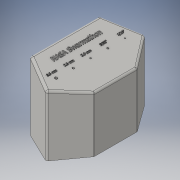
# Autodesk Inventor part: HexKeyStand
Saved by Autodesk Inventor 2016 (Build 200138000, 138)
## iProperties
Created: 2016-07-28
Part Number: HexKeyStand
Material: Generic
Document SubType Name: Modeling
Designer: lachesis
Density: 1 g/cm^3
Appearance: Default
Author: lachesis
Autodesk Inventor part; units mm, degrees
(part 1 of 3)
ref_plane "YZ Plane" through (0, 0, 0) normal (1, 0, 0) x (0, 1, 0)
ref_plane "XZ Plane" through (0, 0, 0) normal (0, 1, 0) x (-1, 0, 0)
ref_plane "XY Plane" through (0, 0, 0) normal (0, 0, 1) x (1, 0, 0)
sketch "Sketch1" plane through (0, 0, 0) normal (0, 1, 0) x (-1, 0, 0)
  line L0 (-29.7389, 31.75) -> (-29.7389, -31.75)
  line L1 (-29.7389, -31.75) -> (0, -72.9354)
  line L2 (0, -72.9354) -> (45.7238, -50.8)
  line L3 (45.7238, -50.8) -> (45.7238, 50.8)
  line L4 (45.7238, 50.8) -> (0, 72.9354)
  line L5 (0, 72.9354) -> (-29.7389, 31.75)
  point P0 (0, 0)
  point P1 (45.7238, 0)
  point P2 (-29.7389, 0)
  dimension "d0" = 101.6
  dimension "d1" = 63.5
  dimension "d2" = 50.8
  dimension "d3" = 50.8
  dimension "d5" = 50.8
  dimension "d6" = 100
  constraints: 12 end point, 2 horizontal alignment, 2 midpoint, 2 vertical alignment, 1 parallel, 1 vertical
  measures "d0" distance of L2.end L3.end
  measures "d1" distance of L0.start L0.end
  measures "d2" distance of L3.end L4.end
  measures "d3" distance of L1.end L2.end
  measures "d5" distance of L4.end L0.start
  measures "d6" angle of L1 L2
extrude "Extrusion1" add sketch "Sketch1" along normal blind 101.6
ref_plane "Work Plane4" through (0, 0, 72.9354) normal (0, 0, -1) x (0, 1, 0)
ref_plane "Work Plane3" through (29.7389, 0, 31.75) normal (0, 0, -1) x (0, 1, 0)
sketch "Sketch3" plane through (0, 0, 72.9354) normal (0, 0, -1) x (0, 1, 0)
  line L0 (0, -45.7238) -> (101.6, -45.7238) projected
  line L1 (101.6, -45.7238) -> (101.6, 0) projected
  line L2 (101.6, 0) -> (101.6, 29.7389) projected
  line L3 (0, 29.7389) -> (101.6, 29.7389) projected
  line L4 (0, -45.7238) -> (101.6, -45.7238) projected
  line L5 (101.6, -45.7238) -> (81.3798, 29.7389)
  point P0 (0, 0)
  dimension "d14" = 15
  constraints: 2 end point, 1 point on line
  measures "d14" angle of L1 L5
extrude "Extrusion3" cut sketch "Sketch3" along normal through all
fillet "Fillet1" radius 3.175 12 edges at (-22.8619, 95.4742, 61.8677) (-45.7238, 101.6, 0) (-45.7238, 50.8, 50.8) (0, 44.6742, 72.9354) (29.7389, 40.6899, 31.75) (14.8695, 85.3641, 52.3427) (29.7389, 81.3798, 0) (29.7389, 40.6899, -31.75) (14.8695, 85.3641, -52.3427) (0, 44.6742, -72.9354) (-22.8619, 95.4742, -61.8677) (-45.7238, 50.8, -50.8)
sketch "Sketch4" plane through (-41.727, 100.5291, 48.8096) normal (0.258819, 0.9659258, 0) x (0.9659258, -0.258819, 0)
  line L0 (0, 0) -> (0, 97.6191) projected
  line L1 (0, 48.8096) -> (71.5508, 48.8096)
  line L2 (71.5508, 79.5331) -> (71.5508, 18.086) projected
  line L3 (35.7754, 48.8096) -> (35.7754, 127.794)
  line L4 (35.7754, 127.794) -> (35.7754, 48.8096)
  line L5 (35.7754, 48.8096) -> (35.7754, -35.2396)
  line L6 (35.7754, 24.8529) -> (37.0254, 24.1313)
  line L7 (37.0254, 24.1313) -> (37.0254, 22.6879)
  line L8 (37.0254, 22.6879) -> (35.7754, 21.9662)
  line L9 (35.7754, 21.9662) -> (34.5254, 22.6879)
  line L10 (34.5254, 22.6879) -> (34.5254, 24.1313)
  line L11 (34.5254, 24.1313) -> (35.7754, 24.8529)
  line L12 (35.7754, 49.9643) -> (36.7754, 49.3869)
  line L13 (36.7754, 49.3869) -> (36.7754, 48.2322)
  line L14 (36.7754, 48.2322) -> (35.7754, 47.6549)
  line L15 (35.7754, 47.6549) -> (34.7754, 48.2322)
  line L16 (34.7754, 48.2322) -> (34.7754, 49.3869)
  line L17 (34.7754, 49.3869) -> (35.7754, 49.9643)
  line L18 (35.7754, 75.5844) -> (36.966, 74.897)
  line L19 (36.966, 74.897) -> (36.966, 73.5222)
  line L20 (36.966, 73.5222) -> (35.7754, 72.8348)
  line L21 (35.7754, 72.8348) -> (34.5848, 73.5222)
  line L22 (34.5848, 73.5222) -> (34.5848, 74.897)
  line L23 (34.5848, 74.897) -> (35.7754, 75.5844)
  line L24 (35.7754, 98.693) -> (34.9816, 99.1513)
  line L25 (34.9816, 99.1513) -> (34.9816, 100.0678)
  line L26 (34.9816, 100.0678) -> (35.7754, 100.5261)
  line L27 (35.7754, 100.5261) -> (36.5691, 100.0678)
  line L28 (36.5691, 100.0678) -> (36.5691, 99.1513)
  line L29 (36.5691, 99.1513) -> (35.7754, 98.693)
  line L30 (35.7754, 0.0303) -> (37.5254, -0.9801)
  line L31 (37.5254, -0.9801) -> (37.5254, -3.0008)
  line L32 (37.5254, -3.0008) -> (35.7754, -4.0112)
  line L33 (35.7754, -4.0112) -> (34.0254, -3.0008)
  line L34 (34.0254, -3.0008) -> (34.0254, -0.9801)
  line L35 (34.0254, -0.9801) -> (35.7754, 0.0303)
  point P0 (66.3241, 48.8096)
  point P1 (35.7754, -1.9904)
  point P2 (35.7754, 23.4096)
  point P3 (35.7754, 74.2096)
  point P4 (35.7754, 99.6096)
  point P5 (35.7754, -1.9904)
  point P6 (35.7754, 23.4096)
  point P7 (35.7754, 74.2096)
  point P8 (35.7754, 99.6096)
  point P9 (35.7754, -1.9904)
  dimension "d18" = 25.4
  dimension "d19" = 25.4
  dimension "d20" = 25.4
  dimension "d22" = 25.4
  dimension "d23" = 3.5
  dimension "d24" = 2.5
  dimension "d25" = 2
  dimension "d26" = 2.3813
  dimension "d27" = 1.5875
  constraints: 68 end point, 9 point on line, 6 coincident, 3 midpoint, 2 vertical, 1 perpendicular, 65 other
  measures "d18" distance of point (35.775, 74.21) L3.start
  measures "d19" distance of point (35.775, 74.21) point (35.775, 99.61)
  measures "d20" distance of L3.start point (35.775, 23.41)
  measures "d22" distance of point (35.775, 23.41) point (35.775, -1.99)
  measures "d23" distance between parallel lines of L31 L34
  measures "d24" distance between parallel lines of L7 L10
  measures "d25" distance between parallel lines of L13 L16
  measures "d26" distance between parallel lines of L19 L22
  measures "d27" distance between parallel lines of L28 L25
extrude "Extrusion4" cut sketch "Sketch4" against normal blind 76.2
sketch "Sketch5" plane through (-41.727, 100.5291, 48.8096) normal (0.258819, 0.9659258, 0) x (0.9659258, -0.258819, 0)
  line L0 (34.0254, -3.0008) -> (34.0254, -0.9801) projected
  spline S0 degree 2 poles (26.7586, -7.3009) (26.7586, -7.412) (26.8129, -7.6319) (26.8549, -7.7381) knots 0 0 0 1 2 2 2
  spline S1 degree 2 poles (26.8549, -7.7381) (26.8969, -7.8369) (26.9858, -7.9826) (27.0254, -8.0394) knots 0 0 0 1 2 2 2
  line L1 (27.0254, -8.0394) -> (27.0254, -8.0641)
  line L2 (27.0254, -8.0641) -> (26.5931, -8.0641)
  spline S2 degree 2 poles (26.5931, -8.0641) (26.5215, -7.9307) (26.4054, -7.4738) (26.4054, -7.2688) knots 0 0 0 1 2 2 2
  spline S3 degree 2 poles (26.4054, -7.2688) (26.4054, -7.0613) (26.4894, -6.7525) (26.5783, -6.6266) knots 0 0 0 1 2 2 2
  spline S4 degree 2 poles (26.5783, -6.6266) (26.6746, -6.4932) (26.9537, -6.3549) (27.1414, -6.3549) knots 0 0 0 1 2 2 2
  spline S5 degree 2 poles (27.1414, -6.3549) (27.3934, -6.3549) (27.7738, -6.6858) (27.8232, -6.918) knots 0 0 0 1 2 2 2
  line L3 (27.8232, -6.918) -> (27.8528, -6.918)
  spline S6 degree 2 poles (27.8528, -6.918) (27.8726, -6.8217) (27.9615, -6.6019) (28.0504, -6.508) knots 0 0 0 1 2 2 2
  spline S7 degree 2 poles (28.0504, -6.508) (28.1369, -6.4141) (28.4135, -6.2956) (28.6136, -6.2956) knots 0 0 0 1 2 2 2
  spline S8 degree 2 poles (28.6136, -6.2956) (28.8186, -6.2956) (29.1669, -6.4364) (29.3002, -6.5648) knots 0 0 0 1 2 2 2
  spline S9 degree 2 poles (29.3002, -6.5648) (29.4386, -6.6982) (29.5818, -7.0761) (29.5818, -7.3157) knots 0 0 0 1 2 2 2
  spline S10 degree 2 poles (29.5818, -7.3157) (29.5818, -7.5454) (29.4707, -7.9949) (29.3941, -8.1481) knots 0 0 0 1 2 2 2
  line L4 (29.3941, -8.1481) -> (28.9619, -8.1481)
  line L5 (28.9619, -8.1481) -> (28.9619, -8.1184)
  spline S11 degree 2 poles (28.9619, -8.1184) (29.0557, -7.99) (29.2286, -7.5553) (29.2286, -7.3404) knots 0 0 0 1 2 2 2
  spline S12 degree 2 poles (29.2286, -7.3404) (29.2286, -7.2144) (29.1496, -6.9625) (29.0582, -6.8785) knots 0 0 0 1 2 2 2
  spline S13 degree 2 poles (29.0582, -6.8785) (28.9668, -6.797) (28.7494, -6.7105) (28.5839, -6.7105) knots 0 0 0 1 2 2 2
  spline S14 degree 2 poles (28.5839, -6.7105) (28.4184, -6.7105) (28.2036, -6.8069) (28.1418, -6.8933) knots 0 0 0 1 2 2 2
  spline S15 degree 2 poles (28.1418, -6.8933) (28.0801, -6.9798) (28.0331, -7.2144) (28.0331, -7.3527) knots 0 0 0 1 2 2 2
  line L6 (28.0331, -7.3527) -> (28.0331, -7.5256)
  line L7 (28.0331, -7.5256) -> (27.6947, -7.5256)
  line L8 (27.6947, -7.5256) -> (27.6947, -7.3898)
  spline S16 degree 2 poles (27.6947, -7.3898) (27.6947, -7.1156) (27.4329, -6.7698) (27.1834, -6.7698) knots 0 0 0 1 2 2 2
  spline S17 degree 2 poles (27.1834, -6.7698) (27.0673, -6.7698) (26.9019, -6.8587) (26.8525, -6.9304) knots 0 0 0 1 2 2 2
  spline S18 degree 2 poles (26.8525, -6.9304) (26.8006, -7.0069) (26.7586, -7.1947) (26.7586, -7.3009) knots 0 0 0 1 2 2 2
  line L9 (29.5176, -5.1816) -> (29.5176, -5.6707)
  line L10 (29.5176, -5.6707) -> (28.9347, -5.6707)
  line L11 (28.9347, -5.6707) -> (28.9347, -5.1816)
  line L12 (28.9347, -5.1816) -> (29.5176, -5.1816)
  spline S19 degree 2 poles (28.5494, -2.719) (28.7692, -2.719) (29.1446, -2.8598) (29.283, -2.9882) knots 0 0 0 1 2 2 2
  spline S20 degree 2 poles (29.283, -2.9882) (29.4213, -3.1167) (29.5818, -3.4995) (29.5818, -3.7366) knots 0 0 0 1 2 2 2
  spline S21 degree 2 poles (29.5818, -3.7366) (29.5818, -3.954) (29.4855, -4.3788) (29.4089, -4.5345) knots 0 0 0 1 2 2 2
  line L13 (29.4089, -4.5345) -> (28.9767, -4.5345)
  line L14 (28.9767, -4.5345) -> (28.9767, -4.5048)
  spline S22 degree 2 poles (28.9767, -4.5048) (29.0113, -4.4579) (29.1002, -4.2825) (29.1397, -4.1763) knots 0 0 0 1 2 2 2
  spline S23 degree 2 poles (29.1397, -4.1763) (29.1817, -4.0553) (29.2286, -3.8552) (29.2286, -3.7292) knots 0 0 0 1 2 2 2
  spline S24 degree 2 poles (29.2286, -3.7292) (29.2286, -3.6057) (29.1397, -3.3735) (29.0434, -3.2896) knots 0 0 0 1 2 2 2
  spline S25 degree 2 poles (29.0434, -3.2896) (28.952, -3.213) (28.7099, -3.134) (28.5469, -3.134) knots 0 0 0 1 2 2 2
  spline S26 degree 2 poles (28.5469, -3.134) (28.3839, -3.134) (28.1764, -3.2229) (28.1072, -3.3069) knots 0 0 0 1 2 2 2
  spline S27 degree 2 poles (28.1072, -3.3069) (28.0307, -3.3933) (27.9664, -3.6502) (27.9664, -3.8058) knots 0 0 0 1 2 2 2
  spline S28 degree 2 poles (27.9664, -3.8058) (27.9664, -3.9738) (28.0183, -4.3072) (28.0405, -4.4085) knots 0 0 0 1 2 2 2
  line L15 (28.0405, -4.4085) -> (26.4696, -4.4085)
  line L16 (26.4696, -4.4085) -> (26.4696, -2.7363)
  line L17 (26.4696, -2.7363) -> (26.8278, -2.7363)
  line L18 (26.8278, -2.7363) -> (26.8278, -4.0158)
  line L19 (26.8278, -4.0158) -> (27.6404, -4.0158)
  spline S29 degree 2 poles (27.6404, -4.0158) (27.6305, -3.9417) (27.6231, -3.7984) (27.6231, -3.7391) knots 0 0 0 1 2 2 2
  spline S30 degree 2 poles (27.6231, -3.7391) (27.6231, -3.5045) (27.6997, -3.1809) (27.8133, -3.0327) knots 0 0 0 1 2 2 2
  spline S31 degree 2 poles (27.8133, -3.0327) (27.9269, -2.882) (28.2727, -2.719) (28.5494, -2.719) knots 0 0 0 1 2 2 2
  line L20 (29.5176, 1.6801) -> (28.1937, 1.6801)
  spline S32 degree 2 poles (28.1937, 1.6801) (28.0356, 1.6801) (27.7664, 1.6554) (27.6923, 1.6159) knots 0 0 0 1 2 2 2
  spline S33 degree 2 poles (27.6923, 1.6159) (27.6108, 1.5764) (27.5317, 1.4257) (27.5317, 1.2948) knots 0 0 0 1 2 2 2
  spline S34 degree 2 poles (27.5317, 1.2948) (27.5317, 1.1762) (27.6774, 0.9045) (27.8158, 0.7613) knots 0 0 0 1 2 2 2
  spline S35 degree 2 poles (27.8158, 0.7613) (27.8503, 0.7637) (27.9467, 0.7687) (28.0109, 0.7687) knots 0 0 0 1 2 2 2
  line L21 (28.0109, 0.7687) -> (29.5176, 0.7687)
  line L22 (29.5176, 0.7687) -> (29.5176, 0.3833)
  line L23 (29.5176, 0.3833) -> (28.1937, 0.3833)
  spline S36 degree 2 poles (28.1937, 0.3833) (28.0356, 0.3833) (27.7664, 0.3586) (27.6923, 0.3191) knots 0 0 0 1 2 2 2
  spline S37 degree 2 poles (27.6923, 0.3191) (27.6108, 0.2796) (27.5317, 0.1289) (27.5317, -0.002) knots 0 0 0 1 2 2 2
  spline S38 degree 2 poles (27.5317, -0.002) (27.5317, -0.1255) (27.6873, -0.3996) (27.8084, -0.5281) knots 0 0 0 1 2 2 2
  line L24 (27.8084, -0.5281) -> (29.5176, -0.5281)
  line L25 (29.5176, -0.5281) -> (29.5176, -0.9134)
  line L26 (29.5176, -0.9134) -> (27.2304, -0.9134)
  line L27 (27.2304, -0.9134) -> (27.2304, -0.5281)
  line L28 (27.2304, -0.5281) -> (27.4823, -0.5281)
  spline S39 degree 2 poles (27.4823, -0.5281) (27.3316, -0.3774) (27.1661, -0.081) (27.1661, 0.0968) knots 0 0 0 1 2 2 2
  spline S40 degree 2 poles (27.1661, 0.0968) (27.1661, 0.2994) (27.3514, 0.6131) (27.5614, 0.6946) knots 0 0 0 1 2 2 2
  spline S41 degree 2 poles (27.5614, 0.6946) (27.3662, 0.8699) (27.1661, 1.2009) (27.1661, 1.3936) knots 0 0 0 1 2 2 2
  spline S42 degree 2 poles (27.1661, 1.3936) (27.1661, 1.5418) (27.2575, 1.7838) (27.3613, 1.8728) knots 0 0 0 1 2 2 2
  spline S43 degree 2 poles (27.3613, 1.8728) (27.465, 1.9642) (27.7762, 2.0654) (28.0109, 2.0654) knots 0 0 0 1 2 2 2
  line L29 (28.0109, 2.0654) -> (29.5176, 2.0654)
  line L30 (29.5176, 2.0654) -> (29.5176, 1.6801)
  line L31 (29.5176, 5.1999) -> (28.1937, 5.1999)
  spline S44 degree 2 poles (28.1937, 5.1999) (28.0356, 5.1999) (27.7664, 5.1752) (27.6923, 5.1357) knots 0 0 0 1 2 2 2
  spline S45 degree 2 poles (27.6923, 5.1357) (27.6108, 5.0961) (27.5317, 4.9455) (27.5317, 4.8146) knots 0 0 0 1 2 2 2
  spline S46 degree 2 poles (27.5317, 4.8146) (27.5317, 4.696) (27.6774, 4.4243) (27.8158, 4.281) knots 0 0 0 1 2 2 2
  spline S47 degree 2 poles (27.8158, 4.281) (27.8503, 4.2835) (27.9467, 4.2884) (28.0109, 4.2884) knots 0 0 0 1 2 2 2
  line L32 (28.0109, 4.2884) -> (29.5176, 4.2884)
  line L33 (29.5176, 4.2884) -> (29.5176, 3.9031)
  line L34 (29.5176, 3.9031) -> (28.1937, 3.9031)
  spline S48 degree 2 poles (28.1937, 3.9031) (28.0356, 3.9031) (27.7664, 3.8784) (27.6923, 3.8389) knots 0 0 0 1 2 2 2
  spline S49 degree 2 poles (27.6923, 3.8389) (27.6108, 3.7994) (27.5317, 3.6487) (27.5317, 3.5178) knots 0 0 0 1 2 2 2
  spline S50 degree 2 poles (27.5317, 3.5178) (27.5317, 3.3943) (27.6873, 3.1201) (27.8084, 2.9917) knots 0 0 0 1 2 2 2
  line L35 (27.8084, 2.9917) -> (29.5176, 2.9917)
  line L36 (29.5176, 2.9917) -> (29.5176, 2.6064)
  line L37 (29.5176, 2.6064) -> (27.2304, 2.6064)
  line L38 (27.2304, 2.6064) -> (27.2304, 2.9917)
  line L39 (27.2304, 2.9917) -> (27.4823, 2.9917)
  spline S51 degree 2 poles (27.4823, 2.9917) (27.3316, 3.1424) (27.1661, 3.4388) (27.1661, 3.6166) knots 0 0 0 1 2 2 2
  spline S52 degree 2 poles (27.1661, 3.6166) (27.1661, 3.8191) (27.3514, 4.1328) (27.5614, 4.2143) knots 0 0 0 1 2 2 2
  spline S53 degree 2 poles (27.5614, 4.2143) (27.3662, 4.3897) (27.1661, 4.7207) (27.1661, 4.9134) knots 0 0 0 1 2 2 2
  spline S54 degree 2 poles (27.1661, 4.9134) (27.1661, 5.0616) (27.2575, 5.3036) (27.3613, 5.3925) knots 0 0 0 1 2 2 2
  spline S55 degree 2 poles (27.3613, 5.3925) (27.465, 5.4839) (27.7762, 5.5852) (28.0109, 5.5852) knots 0 0 0 1 2 2 2
  line L40 (28.0109, 5.5852) -> (29.5176, 5.5852)
  line L41 (29.5176, 5.5852) -> (29.5176, 5.1999)
  line L42 (29.5176, 19.1446) -> (29.5176, 17.2649)
  line L43 (29.5176, 17.2649) -> (29.0854, 17.2649)
  spline S56 degree 2 poles (29.0854, 17.2649) (28.8952, 17.4674) (28.5419, 17.828) (28.3518, 18.001) knots 0 0 0 1 2 2 2
  spline S57 degree 2 poles (28.3518, 18.001) (27.9689, 18.3492) (27.5095, 18.6036) (27.2649, 18.6036) knots 0 0 0 1 2 2 2
  spline S58 degree 2 poles (27.2649, 18.6036) (27.1365, 18.6036) (26.9438, 18.5246) (26.8821, 18.453) knots 0 0 0 1 2 2 2
  spline S59 degree 2 poles (26.8821, 18.453) (26.8203, 18.3813) (26.7586, 18.1936) (26.7586, 18.08) knots 0 0 0 1 2 2 2
  spline S60 degree 2 poles (26.7586, 18.08) (26.7586, 17.9713) (26.8129, 17.749) (26.8549, 17.6477) knots 0 0 0 1 2 2 2
  spline S61 degree 2 poles (26.8549, 17.6477) (26.8895, 17.5613) (26.9883, 17.4007) (27.0229, 17.3513) knots 0 0 0 1 2 2 2
  line L44 (27.0229, 17.3513) -> (27.0229, 17.3291)
  line L45 (27.0229, 17.3291) -> (26.5882, 17.3291)
  spline S62 degree 2 poles (26.5882, 17.3291) (26.5264, 17.4551) (26.4054, 17.9071) (26.4054, 18.1096) knots 0 0 0 1 2 2 2
  spline S63 degree 2 poles (26.4054, 18.1096) (26.4054, 18.5369) (26.8574, 19.0186) (27.2427, 19.0186) knots 0 0 0 1 2 2 2
  spline S64 degree 2 poles (27.2427, 19.0186) (27.423, 19.0186) (27.7244, 18.9346) (27.8528, 18.8605) knots 0 0 0 1 2 2 2
  spline S65 degree 2 poles (27.8528, 18.8605) (27.9862, 18.7864) (28.248, 18.5715) (28.374, 18.453) knots 0 0 0 1 2 2 2
  spline S66 degree 2 poles (28.374, 18.453) (28.5839, 18.2603) (29.0335, 17.7885) (29.1644, 17.6477) knots 0 0 0 1 2 2 2
  line L46 (29.1644, 17.6477) -> (29.1644, 19.1446)
  line L47 (29.1644, 19.1446) -> (29.5176, 19.1446)
  line L48 (29.5176, 20.2067) -> (29.5176, 19.7176)
  line L49 (29.5176, 19.7176) -> (28.9347, 19.7176)
  line L50 (28.9347, 19.7176) -> (28.9347, 20.2067)
  line L51 (28.9347, 20.2067) -> (29.5176, 20.2067)
  spline S67 degree 2 poles (28.5494, 22.6693) (28.7692, 22.6693) (29.1446, 22.5285) (29.283, 22.4) knots 0 0 0 1 2 2 2
  spline S68 degree 2 poles (29.283, 22.4) (29.4213, 22.2716) (29.5818, 21.8888) (29.5818, 21.6516) knots 0 0 0 1 2 2 2
  spline S69 degree 2 poles (29.5818, 21.6516) (29.5818, 21.4343) (29.4855, 21.0094) (29.4089, 20.8538) knots 0 0 0 1 2 2 2
  line L52 (29.4089, 20.8538) -> (28.9767, 20.8538)
  line L53 (28.9767, 20.8538) -> (28.9767, 20.8835)
  spline S70 degree 2 poles (28.9767, 20.8835) (29.0113, 20.9304) (29.1002, 21.1058) (29.1397, 21.212) knots 0 0 0 1 2 2 2
  spline S71 degree 2 poles (29.1397, 21.212) (29.1817, 21.333) (29.2286, 21.5331) (29.2286, 21.659) knots 0 0 0 1 2 2 2
  spline S72 degree 2 poles (29.2286, 21.659) (29.2286, 21.7825) (29.1397, 22.0147) (29.0434, 22.0987) knots 0 0 0 1 2 2 2
  spline S73 degree 2 poles (29.0434, 22.0987) (28.952, 22.1753) (28.7099, 22.2543) (28.5469, 22.2543) knots 0 0 0 1 2 2 2
  spline S74 degree 2 poles (28.5469, 22.2543) (28.3839, 22.2543) (28.1764, 22.1654) (28.1072, 22.0814) knots 0 0 0 1 2 2 2
  spline S75 degree 2 poles (28.1072, 22.0814) (28.0307, 21.995) (27.9664, 21.7381) (27.9664, 21.5825) knots 0 0 0 1 2 2 2
  spline S76 degree 2 poles (27.9664, 21.5825) (27.9664, 21.4145) (28.0183, 21.0811) (28.0405, 20.9798) knots 0 0 0 1 2 2 2
  line L54 (28.0405, 20.9798) -> (26.4696, 20.9798)
  line L55 (26.4696, 20.9798) -> (26.4696, 22.652)
  line L56 (26.4696, 22.652) -> (26.8278, 22.652)
  line L57 (26.8278, 22.652) -> (26.8278, 21.3725)
  line L58 (26.8278, 21.3725) -> (27.6404, 21.3725)
  spline S77 degree 2 poles (27.6404, 21.3725) (27.6305, 21.4466) (27.6231, 21.5899) (27.6231, 21.6492) knots 0 0 0 1 2 2 2
  spline S78 degree 2 poles (27.6231, 21.6492) (27.6231, 21.8838) (27.6997, 22.2074) (27.8133, 22.3556) knots 0 0 0 1 2 2 2
  spline S79 degree 2 poles (27.8133, 22.3556) (27.9269, 22.5063) (28.2727, 22.6693) (28.5494, 22.6693) knots 0 0 0 1 2 2 2
  line L59 (29.5176, 27.0684) -> (28.1937, 27.0684)
  spline S80 degree 2 poles (28.1937, 27.0684) (28.0356, 27.0684) (27.7664, 27.0437) (27.6923, 27.0042) knots 0 0 0 1 2 2 2
  spline S81 degree 2 poles (27.6923, 27.0042) (27.6108, 26.9646) (27.5317, 26.814) (27.5317, 26.6831) knots 0 0 0 1 2 2 2
  spline S82 degree 2 poles (27.5317, 26.6831) (27.5317, 26.5645) (27.6774, 26.2928) (27.8158, 26.1495) knots 0 0 0 1 2 2 2
  spline S83 degree 2 poles (27.8158, 26.1495) (27.8503, 26.152) (27.9467, 26.1569) (28.0109, 26.1569) knots 0 0 0 1 2 2 2
  line L60 (28.0109, 26.1569) -> (29.5176, 26.1569)
  line L61 (29.5176, 26.1569) -> (29.5176, 25.7716)
  line L62 (29.5176, 25.7716) -> (28.1937, 25.7716)
  spline S84 degree 2 poles (28.1937, 25.7716) (28.0356, 25.7716) (27.7664, 25.7469) (27.6923, 25.7074) knots 0 0 0 1 2 2 2
  spline S85 degree 2 poles (27.6923, 25.7074) (27.6108, 25.6679) (27.5317, 25.5172) (27.5317, 25.3863) knots 0 0 0 1 2 2 2
  spline S86 degree 2 poles (27.5317, 25.3863) (27.5317, 25.2628) (27.6873, 24.9886) (27.8084, 24.8602) knots 0 0 0 1 2 2 2
  line L63 (27.8084, 24.8602) -> (29.5176, 24.8602)
  line L64 (29.5176, 24.8602) -> (29.5176, 24.4749)
  line L65 (29.5176, 24.4749) -> (27.2304, 24.4749)
  line L66 (27.2304, 24.4749) -> (27.2304, 24.8602)
  line L67 (27.2304, 24.8602) -> (27.4823, 24.8602)
  spline S87 degree 2 poles (27.4823, 24.8602) (27.3316, 25.0109) (27.1661, 25.3073) (27.1661, 25.4851) knots 0 0 0 1 2 2 2
  spline S88 degree 2 poles (27.1661, 25.4851) (27.1661, 25.6876) (27.3514, 26.0013) (27.5614, 26.0828) knots 0 0 0 1 2 2 2
  spline S89 degree 2 poles (27.5614, 26.0828) (27.3662, 26.2582) (27.1661, 26.5892) (27.1661, 26.7819) knots 0 0 0 1 2 2 2
  spline S90 degree 2 poles (27.1661, 26.7819) (27.1661, 26.9301) (27.2575, 27.1721) (27.3613, 27.261) knots 0 0 0 1 2 2 2
  spline S91 degree 2 poles (27.3613, 27.261) (27.465, 27.3524) (27.7762, 27.4537) (28.0109, 27.4537) knots 0 0 0 1 2 2 2
  line L68 (28.0109, 27.4537) -> (29.5176, 27.4537)
  line L69 (29.5176, 27.4537) -> (29.5176, 27.0684)
  line L70 (29.5176, 30.5882) -> (28.1937, 30.5882)
  spline S92 degree 2 poles (28.1937, 30.5882) (28.0356, 30.5882) (27.7664, 30.5635) (27.6923, 30.5239) knots 0 0 0 1 2 2 2
  spline S93 degree 2 poles (27.6923, 30.5239) (27.6108, 30.4844) (27.5317, 30.3337) (27.5317, 30.2028) knots 0 0 0 1 2 2 2
  spline S94 degree 2 poles (27.5317, 30.2028) (27.5317, 30.0843) (27.6774, 29.8126) (27.8158, 29.6693) knots 0 0 0 1 2 2 2
  spline S95 degree 2 poles (27.8158, 29.6693) (27.8503, 29.6718) (27.9467, 29.6767) (28.0109, 29.6767) knots 0 0 0 1 2 2 2
  line L71 (28.0109, 29.6767) -> (29.5176, 29.6767)
  line L72 (29.5176, 29.6767) -> (29.5176, 29.2914)
  line L73 (29.5176, 29.2914) -> (28.1937, 29.2914)
  spline S96 degree 2 poles (28.1937, 29.2914) (28.0356, 29.2914) (27.7664, 29.2667) (27.6923, 29.2272) knots 0 0 0 1 2 2 2
  spline S97 degree 2 poles (27.6923, 29.2272) (27.6108, 29.1877) (27.5317, 29.037) (27.5317, 28.9061) knots 0 0 0 1 2 2 2
  spline S98 degree 2 poles (27.5317, 28.9061) (27.5317, 28.7826) (27.6873, 28.5084) (27.8084, 28.38) knots 0 0 0 1 2 2 2
  line L74 (27.8084, 28.38) -> (29.5176, 28.38)
  line L75 (29.5176, 28.38) -> (29.5176, 27.9946)
  line L76 (29.5176, 27.9946) -> (27.2304, 27.9946)
  line L77 (27.2304, 27.9946) -> (27.2304, 28.38)
  line L78 (27.2304, 28.38) -> (27.4823, 28.38)
  spline S99 degree 2 poles (27.4823, 28.38) (27.3316, 28.5306) (27.1661, 28.827) (27.1661, 29.0049) knots 0 0 0 1 2 2 2
  spline S100 degree 2 poles (27.1661, 29.0049) (27.1661, 29.2074) (27.3514, 29.5211) (27.5614, 29.6026) knots 0 0 0 1 2 2 2
  spline S101 degree 2 poles (27.5614, 29.6026) (27.3662, 29.778) (27.1661, 30.109) (27.1661, 30.3016) knots 0 0 0 1 2 2 2
  spline S102 degree 2 poles (27.1661, 30.3016) (27.1661, 30.4498) (27.2575, 30.6919) (27.3613, 30.7808) knots 0 0 0 1 2 2 2
  spline S103 degree 2 poles (27.3613, 30.7808) (27.465, 30.8722) (27.7762, 30.9735) (28.0109, 30.9735) knots 0 0 0 1 2 2 2
  line L79 (28.0109, 30.9735) -> (29.5176, 30.9735)
  line L80 (29.5176, 30.9735) -> (29.5176, 30.5882)
  line L81 (29.5176, 44.4508) -> (29.5176, 42.5711)
  line L82 (29.5176, 42.5711) -> (29.0854, 42.5711)
  spline S104 degree 2 poles (29.0854, 42.5711) (28.8952, 42.7737) (28.5419, 43.1343) (28.3518, 43.3072) knots 0 0 0 1 2 2 2
  spline S105 degree 2 poles (28.3518, 43.3072) (27.9689, 43.6554) (27.5095, 43.9099) (27.2649, 43.9099) knots 0 0 0 1 2 2 2
  spline S106 degree 2 poles (27.2649, 43.9099) (27.1365, 43.9099) (26.9438, 43.8308) (26.8821, 43.7592) knots 0 0 0 1 2 2 2
  spline S107 degree 2 poles (26.8821, 43.7592) (26.8203, 43.6876) (26.7586, 43.4998) (26.7586, 43.3862) knots 0 0 0 1 2 2 2
  spline S108 degree 2 poles (26.7586, 43.3862) (26.7586, 43.2775) (26.8129, 43.0552) (26.8549, 42.954) knots 0 0 0 1 2 2 2
  spline S109 degree 2 poles (26.8549, 42.954) (26.8895, 42.8675) (26.9883, 42.707) (27.0229, 42.6576) knots 0 0 0 1 2 2 2
  line L83 (27.0229, 42.6576) -> (27.0229, 42.6353)
  line L84 (27.0229, 42.6353) -> (26.5882, 42.6353)
  spline S110 degree 2 poles (26.5882, 42.6353) (26.5264, 42.7613) (26.4054, 43.2133) (26.4054, 43.4159) knots 0 0 0 1 2 2 2
  spline S111 degree 2 poles (26.4054, 43.4159) (26.4054, 43.8432) (26.8574, 44.3248) (27.2427, 44.3248) knots 0 0 0 1 2 2 2
  spline S112 degree 2 poles (27.2427, 44.3248) (27.423, 44.3248) (27.7244, 44.2408) (27.8528, 44.1667) knots 0 0 0 1 2 2 2
  spline S113 degree 2 poles (27.8528, 44.1667) (27.9862, 44.0926) (28.248, 43.8777) (28.374, 43.7592) knots 0 0 0 1 2 2 2
  spline S114 degree 2 poles (28.374, 43.7592) (28.5839, 43.5665) (29.0335, 43.0948) (29.1644, 42.954) knots 0 0 0 1 2 2 2
  line L85 (29.1644, 42.954) -> (29.1644, 44.4508)
  line L86 (29.1644, 44.4508) -> (29.5176, 44.4508)
  line L87 (29.5176, 45.5129) -> (29.5176, 45.0238)
  line L88 (29.5176, 45.0238) -> (28.9347, 45.0238)
  line L89 (28.9347, 45.0238) -> (28.9347, 45.5129)
  line L90 (28.9347, 45.5129) -> (29.5176, 45.5129)
  spline S115 degree 2 poles (27.9936, 48.0249) (28.8136, 48.0249) (29.5818, 47.5482) (29.5818, 47.0517) knots 0 0 0 1 2 2 2
  spline S116 degree 2 poles (29.5818, 47.0517) (29.5818, 46.5478) (28.7988, 46.0761) (27.9961, 46.0761) knots 0 0 0 1 2 2 2
  spline S117 degree 2 poles (27.9961, 46.0761) (27.1711, 46.0761) (26.4079, 46.5528) (26.4079, 47.0517) knots 0 0 0 1 2 2 2
  spline S118 degree 2 poles (26.4079, 47.0517) (26.4079, 47.5531) (27.1983, 48.0249) (27.9936, 48.0249) knots 0 0 0 1 2 2 2
  spline S119 degree 2 poles (28.9223, 47.5013) (28.7717, 47.5605) (28.3073, 47.6099) (27.9936, 47.6099) knots 0 0 0 1 2 2 2
  spline S120 degree 2 poles (27.9936, 47.6099) (27.6799, 47.6099) (27.218, 47.5605) (27.0624, 47.4988) knots 0 0 0 1 2 2 2
  spline S121 degree 2 poles (27.0624, 47.4988) (26.9068, 47.437) (26.7462, 47.2222) (26.7462, 47.0517) knots 0 0 0 1 2 2 2
  spline S122 degree 2 poles (26.7462, 47.0517) (26.7462, 46.8813) (26.9068, 46.6615) (27.0673, 46.5972) knots 0 0 0 1 2 2 2
  spline S123 degree 2 poles (27.0673, 46.5972) (27.223, 46.5355) (27.6972, 46.491) (27.9961, 46.491) knots 0 0 0 1 2 2 2
  spline S124 degree 2 poles (27.9961, 46.491) (28.3172, 46.491) (28.747, 46.5305) (28.9149, 46.5948) knots 0 0 0 1 2 2 2
  spline S125 degree 2 poles (28.9149, 46.5948) (29.073, 46.654) (29.2434, 46.8739) (29.2434, 47.0517) knots 0 0 0 1 2 2 2
  spline S126 degree 2 poles (29.2434, 47.0517) (29.2434, 47.2197) (29.0829, 47.4395) (28.9223, 47.5013) knots 0 0 0 1 2 2 2
  line L91 (29.5176, 52.3746) -> (28.1937, 52.3746)
  spline S127 degree 2 poles (28.1937, 52.3746) (28.0356, 52.3746) (27.7664, 52.3499) (27.6923, 52.3104) knots 0 0 0 1 2 2 2
  spline S128 degree 2 poles (27.6923, 52.3104) (27.6108, 52.2709) (27.5317, 52.1202) (27.5317, 51.9893) knots 0 0 0 1 2 2 2
  spline S129 degree 2 poles (27.5317, 51.9893) (27.5317, 51.8707) (27.6774, 51.599) (27.8158, 51.4558) knots 0 0 0 1 2 2 2
  spline S130 degree 2 poles (27.8158, 51.4558) (27.8503, 51.4582) (27.9467, 51.4632) (28.0109, 51.4632) knots 0 0 0 1 2 2 2
  line L92 (28.0109, 51.4632) -> (29.5176, 51.4632)
  line L93 (29.5176, 51.4632) -> (29.5176, 51.0778)
  line L94 (29.5176, 51.0778) -> (28.1937, 51.0778)
  spline S131 degree 2 poles (28.1937, 51.0778) (28.0356, 51.0778) (27.7664, 51.0531) (27.6923, 51.0136) knots 0 0 0 1 2 2 2
  spline S132 degree 2 poles (27.6923, 51.0136) (27.6108, 50.9741) (27.5317, 50.8234) (27.5317, 50.6925) knots 0 0 0 1 2 2 2
  spline S133 degree 2 poles (27.5317, 50.6925) (27.5317, 50.569) (27.6873, 50.2949) (27.8084, 50.1664) knots 0 0 0 1 2 2 2
  line L95 (27.8084, 50.1664) -> (29.5176, 50.1664)
  line L96 (29.5176, 50.1664) -> (29.5176, 49.7811)
  line L97 (29.5176, 49.7811) -> (27.2304, 49.7811)
  line L98 (27.2304, 49.7811) -> (27.2304, 50.1664)
  line L99 (27.2304, 50.1664) -> (27.4823, 50.1664)
  spline S134 degree 2 poles (27.4823, 50.1664) (27.3316, 50.3171) (27.1661, 50.6135) (27.1661, 50.7913) knots 0 0 0 1 2 2 2
  spline S135 degree 2 poles (27.1661, 50.7913) (27.1661, 50.9939) (27.3514, 51.3076) (27.5614, 51.3891) knots 0 0 0 1 2 2 2
  spline S136 degree 2 poles (27.5614, 51.3891) (27.3662, 51.5644) (27.1661, 51.8954) (27.1661, 52.0881) knots 0 0 0 1 2 2 2
  spline S137 degree 2 poles (27.1661, 52.0881) (27.1661, 52.2363) (27.2575, 52.4783) (27.3613, 52.5673) knots 0 0 0 1 2 2 2
  spline S138 degree 2 poles (27.3613, 52.5673) (27.465, 52.6587) (27.7762, 52.7599) (28.0109, 52.7599) knots 0 0 0 1 2 2 2
  line L100 (28.0109, 52.7599) -> (29.5176, 52.7599)
  line L101 (29.5176, 52.7599) -> (29.5176, 52.3746)
  line L102 (29.5176, 55.8944) -> (28.1937, 55.8944)
  spline S139 degree 2 poles (28.1937, 55.8944) (28.0356, 55.8944) (27.7664, 55.8697) (27.6923, 55.8302) knots 0 0 0 1 2 2 2
  spline S140 degree 2 poles (27.6923, 55.8302) (27.6108, 55.7906) (27.5317, 55.64) (27.5317, 55.5091) knots 0 0 0 1 2 2 2
  spline S141 degree 2 poles (27.5317, 55.5091) (27.5317, 55.3905) (27.6774, 55.1188) (27.8158, 54.9755) knots 0 0 0 1 2 2 2
  spline S142 degree 2 poles (27.8158, 54.9755) (27.8503, 54.978) (27.9467, 54.9829) (28.0109, 54.9829) knots 0 0 0 1 2 2 2
  line L103 (28.0109, 54.9829) -> (29.5176, 54.9829)
  line L104 (29.5176, 54.9829) -> (29.5176, 54.5976)
  line L105 (29.5176, 54.5976) -> (28.1937, 54.5976)
  spline S143 degree 2 poles (28.1937, 54.5976) (28.0356, 54.5976) (27.7664, 54.5729) (27.6923, 54.5334) knots 0 0 0 1 2 2 2
  spline S144 degree 2 poles (27.6923, 54.5334) (27.6108, 54.4939) (27.5317, 54.3432) (27.5317, 54.2123) knots 0 0 0 1 2 2 2
  spline S145 degree 2 poles (27.5317, 54.2123) (27.5317, 54.0888) (27.6873, 53.8146) (27.8084, 53.6862) knots 0 0 0 1 2 2 2
  line L106 (27.8084, 53.6862) -> (29.5176, 53.6862)
  line L107 (29.5176, 53.6862) -> (29.5176, 53.3009)
  line L108 (29.5176, 53.3009) -> (27.2304, 53.3009)
  line L109 (27.2304, 53.3009) -> (27.2304, 53.6862)
  line L110 (27.2304, 53.6862) -> (27.4823, 53.6862)
  spline S146 degree 2 poles (27.4823, 53.6862) (27.3316, 53.8369) (27.1661, 54.1333) (27.1661, 54.3111) knots 0 0 0 1 2 2 2
  spline S147 degree 2 poles (27.1661, 54.3111) (27.1661, 54.5136) (27.3514, 54.8273) (27.5614, 54.9088) knots 0 0 0 1 2 2 2
  spline S148 degree 2 poles (27.5614, 54.9088) (27.3662, 55.0842) (27.1661, 55.4152) (27.1661, 55.6079) knots 0 0 0 1 2 2 2
  spline S149 degree 2 poles (27.1661, 55.6079) (27.1661, 55.7561) (27.2575, 55.9981) (27.3613, 56.087) knots 0 0 0 1 2 2 2
  spline S150 degree 2 poles (27.3613, 56.087) (27.465, 56.1784) (27.7762, 56.2797) (28.0109, 56.2797) knots 0 0 0 1 2 2 2
  line L111 (28.0109, 56.2797) -> (29.5176, 56.2797)
  line L112 (29.5176, 56.2797) -> (29.5176, 55.8944)
  spline S151 degree 2 poles (26.8302, 71.083) (26.8302, 70.9719) (26.8846, 70.7521) (26.9266, 70.6459) knots 0 0 0 1 2 2 2
  spline S152 degree 2 poles (26.9266, 70.6459) (26.9685, 70.547) (27.0575, 70.4013) (27.097, 70.3445) knots 0 0 0 1 2 2 2
  line L113 (27.097, 70.3445) -> (27.097, 70.3198)
  line L114 (27.097, 70.3198) -> (26.6647, 70.3198)
  spline S153 degree 2 poles (26.6647, 70.3198) (26.5931, 70.4532) (26.477, 70.9101) (26.477, 71.1152) knots 0 0 0 1 2 2 2
  spline S154 degree 2 poles (26.477, 71.1152) (26.477, 71.3226) (26.561, 71.6314) (26.6499, 71.7574) knots 0 0 0 1 2 2 2
  spline S155 degree 2 poles (26.6499, 71.7574) (26.7462, 71.8907) (27.0254, 72.0291) (27.2131, 72.0291) knots 0 0 0 1 2 2 2
  spline S156 degree 2 poles (27.2131, 72.0291) (27.465, 72.0291) (27.8454, 71.6981) (27.8948, 71.4659) knots 0 0 0 1 2 2 2
  line L115 (27.8948, 71.4659) -> (27.9244, 71.4659)
  spline S157 degree 2 poles (27.9244, 71.4659) (27.9442, 71.5622) (28.0331, 71.7821) (28.122, 71.8759) knots 0 0 0 1 2 2 2
  spline S158 degree 2 poles (28.122, 71.8759) (28.2085, 71.9698) (28.4851, 72.0883) (28.6852, 72.0883) knots 0 0 0 1 2 2 2
  spline S159 degree 2 poles (28.6852, 72.0883) (28.8902, 72.0883) (29.2385, 71.9475) (29.3719, 71.8191) knots 0 0 0 1 2 2 2
  spline S160 degree 2 poles (29.3719, 71.8191) (29.5102, 71.6857) (29.6535, 71.3078) (29.6535, 71.0682) knots 0 0 0 1 2 2 2
  spline S161 degree 2 poles (29.6535, 71.0682) (29.6535, 70.8385) (29.5423, 70.389) (29.4657, 70.2358) knots 0 0 0 1 2 2 2
  line L116 (29.4657, 70.2358) -> (29.0335, 70.2358)
  line L117 (29.0335, 70.2358) -> (29.0335, 70.2655)
  spline S162 degree 2 poles (29.0335, 70.2655) (29.1273, 70.3939) (29.3002, 70.8286) (29.3002, 71.0435) knots 0 0 0 1 2 2 2
  spline S163 degree 2 poles (29.3002, 71.0435) (29.3002, 71.1695) (29.2212, 71.4214) (29.1298, 71.5054) knots 0 0 0 1 2 2 2
  spline S164 degree 2 poles (29.1298, 71.5054) (29.0384, 71.5869) (28.8211, 71.6734) (28.6556, 71.6734) knots 0 0 0 1 2 2 2
  spline S165 degree 2 poles (28.6556, 71.6734) (28.4901, 71.6734) (28.2752, 71.577) (28.2134, 71.4906) knots 0 0 0 1 2 2 2
  spline S166 degree 2 poles (28.2134, 71.4906) (28.1517, 71.4041) (28.1048, 71.1695) (28.1048, 71.0312) knots 0 0 0 1 2 2 2
  line L118 (28.1048, 71.0312) -> (28.1048, 70.8583)
  line L119 (28.1048, 70.8583) -> (27.7664, 70.8583)
  line L120 (27.7664, 70.8583) -> (27.7664, 70.9941)
  spline S167 degree 2 poles (27.7664, 70.9941) (27.7664, 71.2683) (27.5045, 71.6141) (27.2551, 71.6141) knots 0 0 0 1 2 2 2
  spline S168 degree 2 poles (27.2551, 71.6141) (27.139, 71.6141) (26.9735, 71.5252) (26.9241, 71.4535) knots 0 0 0 1 2 2 2
  spline S169 degree 2 poles (26.9241, 71.4535) (26.8722, 71.377) (26.8302, 71.1893) (26.8302, 71.083) knots 0 0 0 1 2 2 2
  line L121 (26.4054, 73.8149) -> (30.2512, 72.6219)
  line L122 (30.2512, 72.6219) -> (30.2512, 72.2761)
  line L123 (30.2512, 72.2761) -> (26.4054, 73.4641)
  line L124 (26.4054, 73.4641) -> (26.4054, 73.8149)
  spline S170 degree 2 poles (26.8302, 74.9733) (26.8302, 74.8622) (26.8846, 74.6423) (26.9266, 74.5361) knots 0 0 0 1 2 2 2
  spline S171 degree 2 poles (26.9266, 74.5361) (26.9685, 74.4373) (27.0575, 74.2916) (27.097, 74.2348) knots 0 0 0 1 2 2 2
  line L125 (27.097, 74.2348) -> (27.097, 74.2101)
  line L126 (27.097, 74.2101) -> (26.6647, 74.2101)
  spline S172 degree 2 poles (26.6647, 74.2101) (26.5931, 74.3435) (26.477, 74.8004) (26.477, 75.0054) knots 0 0 0 1 2 2 2
  spline S173 degree 2 poles (26.477, 75.0054) (26.477, 75.2129) (26.561, 75.5217) (26.6499, 75.6476) knots 0 0 0 1 2 2 2
  spline S174 degree 2 poles (26.6499, 75.6476) (26.7462, 75.781) (27.0254, 75.9193) (27.2131, 75.9193) knots 0 0 0 1 2 2 2
  spline S175 degree 2 poles (27.2131, 75.9193) (27.465, 75.9193) (27.8454, 75.5884) (27.8948, 75.3562) knots 0 0 0 1 2 2 2
  line L127 (27.8948, 75.3562) -> (27.9244, 75.3562)
  spline S176 degree 2 poles (27.9244, 75.3562) (27.9442, 75.4525) (28.0331, 75.6723) (28.122, 75.7662) knots 0 0 0 1 2 2 2
  spline S177 degree 2 poles (28.122, 75.7662) (28.2085, 75.8601) (28.4851, 75.9786) (28.6852, 75.9786) knots 0 0 0 1 2 2 2
  spline S178 degree 2 poles (28.6852, 75.9786) (28.8902, 75.9786) (29.2385, 75.8378) (29.3719, 75.7094) knots 0 0 0 1 2 2 2
  spline S179 degree 2 poles (29.3719, 75.7094) (29.5102, 75.576) (29.6535, 75.1981) (29.6535, 74.9585) knots 0 0 0 1 2 2 2
  spline S180 degree 2 poles (29.6535, 74.9585) (29.6535, 74.7288) (29.5423, 74.2792) (29.4657, 74.1261) knots 0 0 0 1 2 2 2
  line L128 (29.4657, 74.1261) -> (29.0335, 74.1261)
  line L129 (29.0335, 74.1261) -> (29.0335, 74.1557)
  spline S181 degree 2 poles (29.0335, 74.1557) (29.1273, 74.2842) (29.3002, 74.7189) (29.3002, 74.9338) knots 0 0 0 1 2 2 2
  spline S182 degree 2 poles (29.3002, 74.9338) (29.3002, 75.0598) (29.2212, 75.3117) (29.1298, 75.3957) knots 0 0 0 1 2 2 2
  spline S183 degree 2 poles (29.1298, 75.3957) (29.0384, 75.4772) (28.8211, 75.5637) (28.6556, 75.5637) knots 0 0 0 1 2 2 2
  spline S184 degree 2 poles (28.6556, 75.5637) (28.4901, 75.5637) (28.2752, 75.4673) (28.2134, 75.3809) knots 0 0 0 1 2 2 2
  spline S185 degree 2 poles (28.2134, 75.3809) (28.1517, 75.2944) (28.1048, 75.0598) (28.1048, 74.9214) knots 0 0 0 1 2 2 2
  line L130 (28.1048, 74.9214) -> (28.1048, 74.7485)
  line L131 (28.1048, 74.7485) -> (27.7664, 74.7485)
  line L132 (27.7664, 74.7485) -> (27.7664, 74.8844)
  spline S186 degree 2 poles (27.7664, 74.8844) (27.7664, 75.1586) (27.5045, 75.5044) (27.2551, 75.5044) knots 0 0 0 1 2 2 2
  spline S187 degree 2 poles (27.2551, 75.5044) (27.139, 75.5044) (26.9735, 75.4155) (26.9241, 75.3438) knots 0 0 0 1 2 2 2
  spline S188 degree 2 poles (26.9241, 75.3438) (26.8722, 75.2673) (26.8302, 75.0795) (26.8302, 74.9733) knots 0 0 0 1 2 2 2
  line L133 (29.5892, 78.3177) -> (29.5892, 76.438)
  line L134 (29.5892, 76.438) -> (29.157, 76.438)
  spline S189 degree 2 poles (29.157, 76.438) (28.9668, 76.6406) (28.6136, 77.0012) (28.4234, 77.1741) knots 0 0 0 1 2 2 2
  spline S190 degree 2 poles (28.4234, 77.1741) (28.0405, 77.5224) (27.5811, 77.7768) (27.3366, 77.7768) knots 0 0 0 1 2 2 2
  spline S191 degree 2 poles (27.3366, 77.7768) (27.2081, 77.7768) (27.0155, 77.6977) (26.9537, 77.6261) knots 0 0 0 1 2 2 2
  spline S192 degree 2 poles (26.9537, 77.6261) (26.892, 77.5545) (26.8302, 77.3668) (26.8302, 77.2531) knots 0 0 0 1 2 2 2
  spline S193 degree 2 poles (26.8302, 77.2531) (26.8302, 77.1445) (26.8846, 76.9222) (26.9266, 76.8209) knots 0 0 0 1 2 2 2
  spline S194 degree 2 poles (26.9266, 76.8209) (26.9611, 76.7344) (27.0599, 76.5739) (27.0945, 76.5245) knots 0 0 0 1 2 2 2
  line L135 (27.0945, 76.5245) -> (27.0945, 76.5023)
  line L136 (27.0945, 76.5023) -> (26.6598, 76.5023)
  spline S195 degree 2 poles (26.6598, 76.5023) (26.598, 76.6282) (26.477, 77.0802) (26.477, 77.2828) knots 0 0 0 1 2 2 2
  spline S196 degree 2 poles (26.477, 77.2828) (26.477, 77.7101) (26.929, 78.1918) (27.3144, 78.1918) knots 0 0 0 1 2 2 2
  spline S197 degree 2 poles (27.3144, 78.1918) (27.4947, 78.1918) (27.796, 78.1078) (27.9244, 78.0337) knots 0 0 0 1 2 2 2
  spline S198 degree 2 poles (27.9244, 78.0337) (28.0578, 77.9596) (28.3196, 77.7447) (28.4456, 77.6261) knots 0 0 0 1 2 2 2
  spline S199 degree 2 poles (28.4456, 77.6261) (28.6556, 77.4335) (29.1051, 76.9617) (29.236, 76.8209) knots 0 0 0 1 2 2 2
  line L137 (29.236, 76.8209) -> (29.236, 78.3177)
  line L138 (29.236, 78.3177) -> (29.5892, 78.3177)
  line L139 (26.4054, 79.9529) -> (27.591, 79.864)
  line L140 (27.591, 79.864) -> (27.591, 79.5947)
  line L141 (27.591, 79.5947) -> (26.4054, 79.5058)
  line L142 (26.4054, 79.5058) -> (26.4054, 79.9529)
  line L143 (26.4054, 79.1822) -> (27.591, 79.0933)
  line L144 (27.591, 79.0933) -> (27.591, 78.8241)
  line L145 (27.591, 78.8241) -> (26.4054, 78.7352)
  line L146 (26.4054, 78.7352) -> (26.4054, 79.1822)
  line L147 (29.5892, 97.6942) -> (29.5892, 96.2073)
  line L148 (29.5892, 96.2073) -> (29.278, 96.2073)
  line L149 (29.278, 96.2073) -> (29.278, 96.7605)
  line L150 (29.278, 96.7605) -> (27.2353, 96.7605)
  line L151 (27.2353, 96.7605) -> (27.2353, 96.2073)
  line L152 (27.2353, 96.2073) -> (26.9562, 96.2073)
  spline S200 degree 2 poles (26.9562, 96.2073) (26.9562, 96.5209) (26.7784, 96.8173) (26.5314, 96.8371) knots 0 0 0 1 2 2 2
  line L153 (26.5314, 96.8371) -> (26.5314, 97.1533)
  line L154 (26.5314, 97.1533) -> (29.278, 97.1533)
  line L155 (29.278, 97.1533) -> (29.278, 97.6942)
  line L156 (29.278, 97.6942) -> (29.5892, 97.6942)
  line L157 (26.4054, 99.522) -> (30.2512, 98.329)
  line L158 (30.2512, 98.329) -> (30.2512, 97.9832)
  line L159 (30.2512, 97.9832) -> (26.4054, 99.1713)
  line L160 (26.4054, 99.1713) -> (26.4054, 99.522)
  line L161 (29.5892, 101.5845) -> (29.5892, 100.0975)
  line L162 (29.5892, 100.0975) -> (29.278, 100.0975)
  line L163 (29.278, 100.0975) -> (29.278, 100.6508)
  line L164 (29.278, 100.6508) -> (27.2353, 100.6508)
  line L165 (27.2353, 100.6508) -> (27.2353, 100.0975)
  line L166 (27.2353, 100.0975) -> (26.9562, 100.0975)
  spline S201 degree 2 poles (26.9562, 100.0975) (26.9562, 100.4112) (26.7784, 100.7076) (26.5314, 100.7274) knots 0 0 0 1 2 2 2
  line L167 (26.5314, 100.7274) -> (26.5314, 101.0435)
  line L168 (26.5314, 101.0435) -> (29.278, 101.0435)
  line L169 (29.278, 101.0435) -> (29.278, 101.5845)
  line L170 (29.278, 101.5845) -> (29.5892, 101.5845)
  spline S202 degree 2 poles (28.6012, 104.0718) (28.8359, 104.0718) (29.2336, 103.9162) (29.3669, 103.7853) knots 0 0 0 1 2 2 2
  spline S203 degree 2 poles (29.3669, 103.7853) (29.5077, 103.6494) (29.6535, 103.3086) (29.6535, 103.1035) knots 0 0 0 1 2 2 2
  spline S204 degree 2 poles (29.6535, 103.1035) (29.6535, 102.8985) (29.5151, 102.5601) (29.3768, 102.4317) knots 0 0 0 1 2 2 2
  spline S205 degree 2 poles (29.3768, 102.4317) (29.2113, 102.2736) (28.6556, 102.0958) (28.2505, 102.0958) knots 0 0 0 1 2 2 2
  spline S206 degree 2 poles (28.2505, 102.0958) (27.8528, 102.0958) (27.2131, 102.2588) (26.976, 102.4292) knots 0 0 0 1 2 2 2
  spline S207 degree 2 poles (26.976, 102.4292) (26.7438, 102.5947) (26.4844, 103.1184) (26.4844, 103.4617) knots 0 0 0 1 2 2 2
  spline S208 degree 2 poles (26.4844, 103.4617) (26.4844, 103.563) (26.5042, 103.7408) (26.5264, 103.8075) knots 0 0 0 1 2 2 2
  line L171 (26.5264, 103.8075) -> (26.9191, 103.8075)
  line L172 (26.9191, 103.8075) -> (26.9191, 103.7902)
  spline S209 degree 2 poles (26.9191, 103.7902) (26.8895, 103.7334) (26.8376, 103.5259) (26.8376, 103.4074) knots 0 0 0 1 2 2 2
  spline S210 degree 2 poles (26.8376, 103.4074) (26.8376, 103.027) (27.3514, 102.5601) (27.8553, 102.5157) knots 0 0 0 1 2 2 2
  spline S211 degree 2 poles (27.8553, 102.5157) (27.754, 102.6614) (27.6429, 102.9677) (27.6429, 103.1505) knots 0 0 0 1 2 2 2
  spline S212 degree 2 poles (27.6429, 103.1505) (27.6429, 103.3283) (27.7145, 103.5951) (27.8232, 103.7408) knots 0 0 0 1 2 2 2
  spline S213 degree 2 poles (27.8232, 103.7408) (27.9491, 103.9088) (28.3394, 104.0718) (28.6012, 104.0718) knots 0 0 0 1 2 2 2
  spline S214 degree 2 poles (28.6185, 103.6568) (28.4308, 103.6568) (28.1764, 103.558) (28.0875, 103.4493) knots 0 0 0 1 2 2 2
  spline S215 degree 2 poles (28.0875, 103.4493) (28.0232, 103.3678) (27.9813, 103.1653) (27.9813, 103.0591) knots 0 0 0 1 2 2 2
  spline S216 degree 2 poles (27.9813, 103.0591) (27.9813, 102.9158) (28.0677, 102.6466) (28.1492, 102.5157) knots 0 0 0 1 2 2 2
  spline S217 degree 2 poles (28.1492, 102.5157) (28.1937, 102.5132) (28.2777, 102.5083) (28.3419, 102.5083) knots 0 0 0 1 2 2 2
  spline S218 degree 2 poles (28.3419, 102.5083) (28.658, 102.5083) (29.0458, 102.6318) (29.1471, 102.7256) knots 0 0 0 1 2 2 2
  spline S219 degree 2 poles (29.1471, 102.7256) (29.2434, 102.8121) (29.32, 102.9998) (29.32, 103.106) knots 0 0 0 1 2 2 2
  spline S220 degree 2 poles (29.32, 103.106) (29.32, 103.353) (28.9693, 103.6568) (28.6185, 103.6568) knots 0 0 0 1 2 2 2
  line L173 (26.4054, 104.8894) -> (27.591, 104.8004)
  line L174 (27.591, 104.8004) -> (27.591, 104.5312)
  line L175 (27.591, 104.5312) -> (26.4054, 104.4423)
  line L176 (26.4054, 104.4423) -> (26.4054, 104.8894)
  line L177 (26.4054, 105.66) -> (27.591, 105.5711)
  line L178 (27.591, 105.5711) -> (27.591, 105.3019)
  line L179 (27.591, 105.3019) -> (26.4054, 105.2129)
  line L180 (26.4054, 105.2129) -> (26.4054, 105.66)
  point P0 (66.3241, 48.8096)
  point P1 (26.4054, -8.3457)
  point P2 (26.4054, 17.0426)
  point P3 (26.4054, 42.3488)
  point P4 (26.4054, 70.0382)
  point P5 (26.4054, 95.7454)
  dimension "d30" = 7.62
  constraints: 4 vertical alignment, 5 other
  measures "d30" distance from line of L0 point (26.405, -8.346)
extrude "Extrusion5" add sketch "Sketch5" along normal blind 1.27